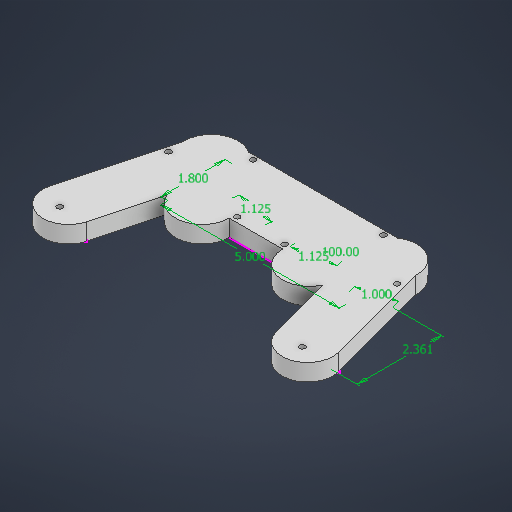
# Autodesk Inventor part: frame
Saved by Autodesk Inventor 2026.2 (Build 302298000, 298)
## iProperties
Created: 2025-12-27
Part Number: frame
Material: Generic
Document SubType Name: Modeling
Designer: Koda
Density: 1 g/cm^3
Appearance: Default
Author: Koda
Autodesk Inventor part; units mm, degrees
ref_plane "YZ Plane" through (0, 0, 0) normal (1, 0, 0) x (0, 1, 0)
ref_plane "XZ Plane" through (0, 0, 0) normal (0, 1, 0) x (-1, 0, 0)
ref_plane "XY Plane" through (0, 0, 0) normal (0, 0, 1) x (1, 0, 0)
sketch "Sketch1" plane through (0, 0, 0) normal (0, 1, 0) x (-1, 0, 0)
  line L0 (0, 0) -> (63.5, 0)
  line L1 (0, 0) -> (-63.5, 0)
  line L2 (0, 0) -> (0, 31.75)
  line L3 (0, 31.75) -> (38.1, 31.75)
  line L4 (0, 31.75) -> (-38.1, 31.75)
  circle A0 centre (38.1, 31.75) radius 15.875
  circle A1 centre (-38.1, 31.75) radius 15.875
  circle A2 centre (63.5, 0) radius 15.875
  circle A3 centre (-63.5, 0) radius 15.875
  circle A4 centre (63.5, 0) radius 19.05
  circle A5 centre (38.1, 31.75) radius 19.05
  circle A6 centre (-38.1, 31.75) radius 19.05
  circle A7 centre (-63.5, 0) radius 19.05
  line L5 (52.9697, -15.875) -> (-52.9697, -15.875)
  line L6 (79.375, -10.5303) -> (102.384, 75.3405)
  line L7 (79.375, -10.5303) -> (168.275, -10.5303) construction
  line L8 (-79.375, -10.5303) -> (-102.384, 75.3405)
  line L9 (-79.375, -10.5303) -> (9.525, -10.5303) construction
  line L10 (63.5, 0) -> (84.9399, 80.0147)
  line L11 (-63.5, 0) -> (-84.9399, 80.0147)
  circle A8 centre (84.9399, 80.0147) radius 18.0595
  circle A9 centre (-84.9399, 80.0147) radius 18.0595
  line L12 (67.4957, 84.6888) -> (55.4302, 39.6598)
  line L13 (-67.4957, 84.6888) -> (-55.4302, 39.6598)
  point P0 (19.05, 31.75)
  point P1 (-19.05, 31.75)
  point P2 (-82.5133, 1.182)
  point P3 (82.5133, 1.182)
  dimension "d10" = 38.1
  dimension "d11" = 38.1
  dimension "d0" = 63.5
  dimension "d1" = 63.5
  dimension "d2" = 31.75
  dimension "d3" = 38.1
  dimension "d4" = 38.1
  dimension "d5" = 31.75
  dimension "d6" = 31.75
  dimension "d7" = 31.75
  dimension "d8" = 31.75
  dimension "d9" = 38.1
  dimension "d12" = 38.1
  dimension "d13" = 88.9
  dimension "d14" = 75
  dimension "d15" = 88.9
  dimension "d16" = 105
  dimension "d17" = 47.625
  constraints: 28 end point, 10 coincident, 8 centre point, 8 point on circle, 6 horizontal, 2 equal length, 2 tangent, 1 parallel, 1 perpendicular, 1 vertical, 6 other
  measures "d0" distance of L0.start L0.end
  measures "d1" distance of L0.start L1.end
  measures "d2" distance of L0.start L2.end
  measures "d3" distance of L2.end L3.end
  measures "d4" distance of L2.end L4.end
  measures "d5" diameter of A0
  measures "d6" diameter of A1
  measures "d7" diameter of A2
  measures "d8" diameter of A3
  measures "d9" diameter of A4
  measures "d12" diameter of A7
  measures "d13" distance of L6.start L6.end
  measures "d14" angle of L7 L6
  measures "d15" distance of L8.start L8.end
  measures "d16" angle of L9 L8
  measures "d17" distance between parallel lines of L3 L5
ref_plane "Work Plane6" through (0, 0, 0) normal (0, -1, 0) x (1, 0, 0)
sketch "Sketch2" plane through (0, 0, 0) normal (0, -1, 0) x (1, 0, 0)
  line L0 (63.5, -14.9037) -> (-63.5, -14.9037)
  line L1 (-63.5, -14.9037) -> (-63.5, 30.8163)
  line L2 (-63.5, 30.8163) -> (63.5, 30.8163)
  line L3 (63.5, 30.8163) -> (63.5, -14.9037)
  point P0 (0, 0)
  dimension "d28" = 127
  dimension "d29" = 45.72
  constraints: 8 end point, 2 parallel, 1 horizontal, 1 perpendicular
  measures "d28" distance of L1.end L2.end
  measures "d29" distance of L0.end L1.end
ref_plane "Work Plane5" through (0, 0, 0) normal (0, -1, 0) x (1, 0, 0)
sketch "Sketch3" plane through (0, 0, 0) normal (0, -1, 0) x (1, 0, 0)
  line L0 (102.384, 75.3405) -> (87.0499, 79.4493) projected
  line L1 (97.893, 76.5439) -> (81.8212, 16.5629)
  line L2 (81.8212, 16.5629) -> (57.2867, 23.1369)
  line L3 (57.2867, 23.1369) -> (73.3585, 83.1179)
  line L4 (67.4957, 84.6888) -> (82.8298, 80.5801) projected
  line L5 (97.893, 76.5439) -> (73.3585, 83.1179)
  point P0 (0, 0)
  dimension "d32" = 25.4
  dimension "d36" = 59.981
  constraints: 8 end point, 3 perpendicular, 2 point on line, 1 collinear
  measures "d32" distance of L1.end L2.end
  measures "d36" vertical distance of L1.start L1.end
ref_plane "Work Plane4" through (0, 0, 0) normal (0, -1, 0) x (1, 0, 0)
sketch "Sketch4" plane through (0, 0, 0) normal (0, -1, 0) x (1, 0, 0)
  line L0 (-102.384, 75.3405) -> (-87.0499, 79.4493) projected
  line L1 (-98.2237, 76.4553) -> (-82.1781, 16.5723)
  line L2 (-82.1781, 16.5723) -> (-57.6862, 23.1349)
  line L3 (-57.6862, 23.1349) -> (-73.7318, 83.0179)
  line L4 (-67.4957, 84.6888) -> (-82.8298, 80.5801) projected
  line L5 (-98.2237, 76.4553) -> (-73.7318, 83.0179)
  point P0 (0, 0)
  constraints: 8 end point, 4 perpendicular, 2 point on line
ref_plane "Work Plane3" through (0, 0, 0) normal (0, -1, 0) x (1, 0, 0)
sketch "Sketch5" plane through (0, 0, 0) normal (0, -1, 0) x (1, 0, 0)
  circle A0 centre (86.2014, 84.9766) radius 2
  circle A1 centre (-86.1442, 84.9766) radius 2
  circle A2 centre (81.1376, 12.5093) radius 2
  circle A3 centre (-81.3994, 12.5093) radius 2
  circle A4 centre (16.8184, 28.0713) radius 2
  circle A5 centre (-16.9553, 28.0713) radius 2
  circle A6 centre (46.1554, -12.6643) radius 2
  circle A7 centre (-46.3495, -12.6643) radius 2
  point P0 (0, 0)
  dimension "d40" = 4
  dimension "d41" = 4
  dimension "d42" = 4
  dimension "d43" = 4
  dimension "d44" = 4
  dimension "d45" = 4
  dimension "d46" = 4
  dimension "d47" = 4
  constraints: 8 centre point
  measures "d40" diameter of A0
  measures "d41" diameter of A1
  measures "d42" diameter of A2
  measures "d43" diameter of A3
  measures "d44" diameter of A4
  measures "d45" diameter of A5
  measures "d46" diameter of A6
  measures "d47" diameter of A7
ref_plane "Work Plane1" through (0, 3.175, 0) normal (0, -1, 0) x (1, 0, 0)
sketch "Sketch6" plane through (0, 3.175, 0) normal (0, -1, 0) x (1, 0, 0)
  line L0 (38.8764, -14.4554) -> (38.8764, 9.5053)
  line L1 (38.8764, 9.5053) -> (10.7355, 14.4673)
  line L2 (10.7355, 14.4673) -> (10.7355, 29.9618)
  line L3 (10.7355, 29.9618) -> (-11.0414, 29.9618)
  line L4 (-11.0414, 29.9618) -> (-11.0414, 14.4673)
  line L5 (-11.0414, 14.4673) -> (-39.1823, 9.5053)
  line L6 (-39.1823, 9.5053) -> (-39.1823, -14.4554)
  line L7 (-39.1823, -14.4554) -> (38.8764, -14.4554)
  line L8 (38.8764, -14.4554) -> (-39.1823, -14.4554)
  line L9 (38.8764, -14.4554) -> (-39.1823, -14.4554)
  line L10 (58.0324, -14.9037) -> (-58.0324, -14.9037) projected
  line L11 (38.8764, -13.9) -> (-39.1823, -13.9)
  line L12 (10.7355, 14.4673) -> (-11.0414, 14.4673)
  point P0 (0, 0)
  dimension "d50" = 28.575
  dimension "d51" = 100
  dimension "d52" = 28.575
  constraints: 24 end point, 5 perpendicular, 4 parallel, 2 point on line, 1 vertical
  measures "d50" distance of L0.end L1.end
  measures "d51" angle of L1 L0
  measures "d52" distance of L4.end L5.end
ref_plane "Work Plane2" through (0, 0, 0) normal (0, -1, 0) x (1, 0, 0)
sketch "Sketch7" plane through (0, 0, 0) normal (0, -1, 0) x (1, 0, 0)
  line L0 (38.9176, -14.5124) -> (38.9176, 9.5046)
  line L1 (38.9176, 9.5046) -> (10.75, 14.4711)
  line L2 (10.75, 14.4711) -> (10.75, 29.8615)
  line L3 (-53.975, 30.8163) -> (22.225, 30.8163) projected
  line L4 (10.75, 29.8615) -> (-10.985, 29.8615)
  line L5 (-10.985, 29.8615) -> (-10.985, 14.4711)
  line L6 (-10.985, 14.4711) -> (-39.3551, 9.5046)
  line L7 (-39.3551, 9.5046) -> (-39.3551, -14.5124)
  line L8 (-39.3551, -14.5124) -> (38.9176, -14.5124)
  point P0 (0, 0)
  point P1 (-53.975, 31.75)
  point P2 (22.225, 31.75)
  constraints: 16 end point, 4 perpendicular, 1 parallel, 1 vertical
extrude "Extrusion7" add sketch "Sketch1" along normal blind 12 contours L2 L3 A5 L12 A8 L10 A4 L0 | L0 A4 L5 A7 L1 | L1 A7 L11 A9 L13 A6 L4 L2 | A4 L10 A2 L0 | L0 A2 L10 A4 L6 | A7 L8 L11 A3 L1 | L1 A3 L11 A7 | A2 L10 L0 | L0 L10 A2 | L10 A8 L6 A4 | A3 L11 L1 | L1 L11 A3 | A7 L8 A9 L11 | A5 | A6 | A4 L6 | A8 | A7 L8 | A9 | A0 | A1
extrude "Extrusion8" cut sketch "Sketch5" against normal blind 19.05
body "Solid2"
